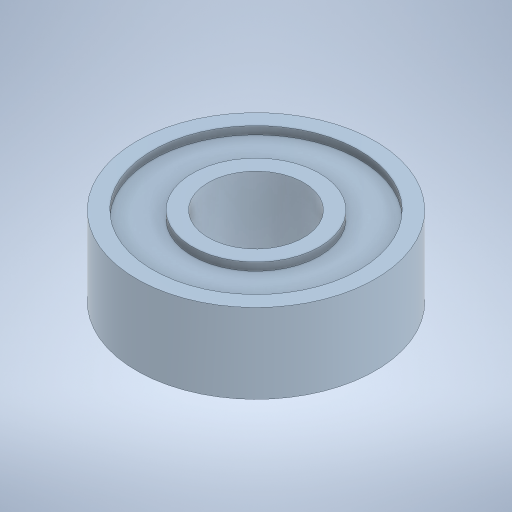
# Autodesk Inventor part: bearing_d6D15b5
Saved by Autodesk Inventor 2023.1 (Build 271208000, 208)
## iProperties
Created: 2023-11-21
Part Number: bearing_d6D15b5
Material: Generic
Document SubType Name: Modeling
Designer: zavrel
Density: 1 g/cm^3
Appearance: Steel Blue
Author: zavrel
Autodesk Inventor part; units mm, degrees
ref_plane "YZ Plane" through (0, 0, 0) normal (1, 0, 0) x (0, 1, 0)
ref_plane "XZ Plane" through (0, 0, 0) normal (0, 1, 0) x (-1, 0, 0)
ref_plane "XY Plane" through (0, 0, 0) normal (0, 0, 1) x (1, 0, 0)
sketch "Sketch1" plane through (0, 0, 0) normal (0, 1, 0) x (-1, 0, 0)
  circle A0 centre (0, 0) radius 7.5
  circle A1 centre (0, 0) radius 3
  dimension "d0" = 6
  dimension "d1" = 15
  constraints: 2 centre point, 2 coincident
  measures "d0" diameter of A1
  measures "d1" diameter of A0
extrude "Extrusion1" add sketch "Sketch1" along normal blind 5
sketch "Sketch2" plane through (0, 5, 0) normal (0, 1, 0) x (1, 0, 0)
  circle A0 centre (0, 0) radius 7.5 projected
  circle A1 centre (0, 0) radius 3 projected
  circle A2 centre (0, 0) radius 3 projected
  circle A3 centre (0, 0) radius 6.5
  circle A4 centre (0, 0) radius 4
  dimension "d4" = 1
  dimension "d5" = 1
  constraints: 2 centre point, 2 coincident
  measures "d4" radial gap between concentric circles of A0 A3
  measures "d5" radial gap between concentric circles of A1 A4
extrude "Extrusion2" cut sketch "Sketch2" against normal blind 0.5 contours A3
sketch "Sketch3" plane through (0, 0, 0) normal (0, -1, 0) x (1, 0, 0)
  circle A0 centre (0, 0) radius 7.5 projected
  circle A1 centre (0, 0) radius 3 projected
  circle A2 centre (0, 0) radius 4
  circle A3 centre (0, 0) radius 6.5
  dimension "d8" = 1
  dimension "d9" = 1
  constraints: 2 centre point, 2 coincident
  measures "d8" radial gap between concentric circles of A0 A3
  measures "d9" radial gap between concentric circles of A1 A2
extrude "Extrusion3" cut sketch "Sketch3" against normal blind 0.5 contours A3
body "Solid1"
